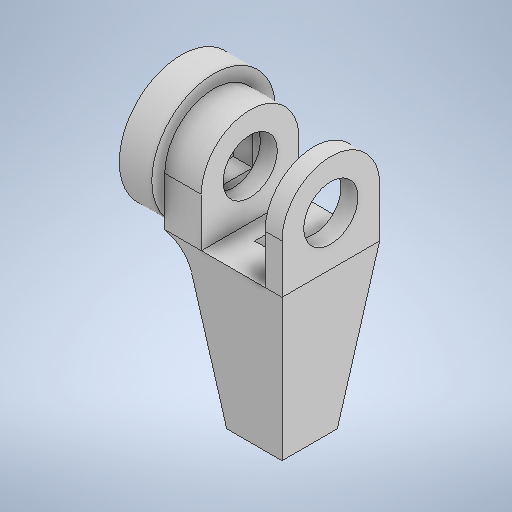
# Autodesk Inventor part: Hip joint 4 med servofeste
Saved by Autodesk Inventor 2025.1 (Build 291241020, 241B)
## iProperties
Created: 2024-10-28
Part Number: Hip joint 4 med servofeste
Material: Generic
Document SubType Name: Modeling
Designer: morte
Density: 1 g/cm^3
Appearance: Default
Author: morte
Autodesk Inventor part; units mm, degrees
ref_plane "YZ Plane" through (0, 0, 0) normal (1, 0, 0) x (0, 1, 0)
ref_plane "XZ Plane" through (0, 0, 0) normal (0, 1, 0) x (-1, 0, 0)
ref_plane "XY Plane" through (0, 0, 0) normal (0, 0, 1) x (1, 0, 0)
sketch "Sketch1" plane through (0, 0, 0) normal (0, 0, 1) x (1, 0, 0)
  line L0 (0, 0) -> (-7.5, 0)
  line L1 (-7.5, 0) -> (-7.5, 15)
  line L2 (-7.5, 15) -> (7.5, 15)
  line L3 (7.5, 15) -> (7.5, 0)
  line L4 (7.5, 0) -> (-7.5, 0)
  dimension "d55" = 7.5
  dimension "d56" = 15
  dimension "d57" = 15
  constraints: 10 end point, 4 perpendicular, 1 horizontal, 1 point on line
  measures "d55" distance of L0.start L0.end
  measures "d56" distance of L0.end L1.end
  measures "d57" distance of L1.end L2.end
extrude "Extrusion1" add sketch "Sketch1" along normal mid plane 15
sketch "Sketch11" plane through (0, 0, 7.5) normal (0, 0, 1) x (1, 0, 0)
  line L0 (7.5, 15) -> (-7.5, 15) projected
  line L1 (0, 15) -> (0, -25)
  line L2 (0, -25) -> (4.25, -25)
  line L3 (0, -25) -> (-4.25, -25)
  line L4 (-7.5, 0) -> (7.5, 0) projected
  line L5 (-4.25, -25) -> (-7.5, 0)
  line L6 (-7.5, 0) -> (7.5, 0)
  line L7 (7.5, 0) -> (4.25, -25)
  point P0 (0, 0)
  dimension "d58" = 40
  dimension "d59" = 4.25
  dimension "d60" = 4.25
  constraints: 12 end point, 2 horizontal, 1 midpoint, 1 parallel, 1 vertical
  measures "d58" distance of L1.start L1.end
  measures "d59" distance of L1.end L2.end
  measures "d60" distance of L1.end L3.end
extrude "Extrusion7" add sketch "Sketch11" against normal blind 15
sketch "Sketch13" plane through (0, 0, 0) normal (1, 0, 0) x (0, 1, 0)
  line L0 (15, -7.5) -> (15, 7.5) projected
  line L1 (15, 0) -> (-25, 0)
  line L2 (-25, 7.5) -> (-25, -7.5) projected
  line L3 (-25, 0) -> (-25, 4.25)
  line L4 (-25, 7.5) -> (-25, -7.5) projected
  line L5 (-25, 4.25) -> (-25, 0)
  line L6 (-25, 0) -> (-25, -4.25)
  line L7 (0, -7.5) -> (15, -7.5) projected
  line L8 (-25, -4.25) -> (0, -7.5)
  line L9 (0, -7.5) -> (0, 7.5)
  line L10 (0, 7.5) -> (-25, 4.25)
  line L11 (-25, 4.25) -> (-25, 7.5)
  line L12 (-25, 7.5) -> (0, 7.5)
  line L13 (-25, -4.25) -> (-25, -7.5)
  line L14 (-25, -7.5) -> (0, -7.5) projected
  line L15 (-25, -7.5) -> (0, -7.5)
  point P0 (0, 0)
  dimension "d68" = 40
  dimension "d69" = 4.25
  dimension "d70" = 4.25
  constraints: 22 end point, 4 collinear, 2 midpoint, 2 point on line, 1 parallel, 1 perpendicular
  measures "d68" distance of L1.start L1.end
  measures "d69" distance of L1.end L3.end
  measures "d70" distance of L1.end L6.end
extrude "Extrusion8" cut sketch "Sketch13" along normal through all both and the other way through all contours L14 L2 L8 | L10 L2 L12
sketch "Sketch15" plane through (-4.25, -25, -4.25) normal (0, -1, 0) x (1, 0, 0)
  line L0 (4.25, 4.25) -> (2.15, 4.25)
  line L1 (0, 8.5) -> (0, 0) projected
  line L2 (2.15, 4.25) -> (2.15, 2.15)
  line L3 (2.15, 2.15) -> (6.35, 2.15)
  line L4 (6.35, 2.15) -> (6.35, 6.35)
  line L5 (6.35, 6.35) -> (2.15, 6.35)
  line L6 (2.15, 6.35) -> (2.15, 4.25)
  point P0 (8.5, 8.5)
  point P1 (8.5, 0)
  dimension "d112" = 2.1
  dimension "d113" = 2.1
  dimension "d114" = 4.2
  dimension "d115" = 4.2
  constraints: 12 end point, 6 perpendicular, 1 point on line
  measures "d112" distance of L0.start L0.end
  measures "d113" distance of L0.end L2.end
  measures "d114" distance of L2.end L3.end
  measures "d115" distance of L3.end L4.end
extrude "Extrusion9" cut sketch "Sketch15" against normal through all
sketch "Sketch16" plane through (0, 0, 7.5) normal (0, 0, 1) x (1, 0, 0)
  line L0 (0, 0) -> (4.9, 0)
  line L1 (-7.5, 0) -> (7.5, 0) projected
  line L2 (4.9, 0) -> (4.9, 16.5506)
  line L3 (0, 0) -> (-4.9, 0)
  line L4 (-4.9, 0) -> (-4.9, 16.5506)
  line L5 (-4.9, 16.5506) -> (4.9, 16.5506)
  dimension "d83" = 4.9
  dimension "d84" = 4.9
  constraints: 10 end point, 2 perpendicular, 2 point on line, 1 vertical
  measures "d83" distance of L0.start L0.end
  measures "d84" distance of L0.start L3.end
extrude "Extrusion10" cut sketch "Sketch16" against normal through all
sketch "Sketch17" plane through (7.5, 15, 7.5) normal (1, 0, 0) x (0, 0, -1)
  line L0 (15, 0) -> (0, 0) projected
  line L1 (0, 0) -> (7.5, 0)
  line L2 (0, 0) -> (0, -15) projected
  line L3 (0, -7.5) -> (0, 0)
  line L4 (0, 0) -> (15, 0)
  line L5 (15, -15) -> (15, 0) projected
  line L6 (15, 0) -> (15, -7.5)
  arc A0 (15, -7.5) -> (0, -7.5) centre (7.5, -7.5) ccw
  line L7 (0, -15) -> (0, 0) projected
  line L8 (0, -7.5) -> (0, 0)
  line L9 (15, 0) -> (0, 0) projected
  line L10 (0, 0) -> (15, 0)
  line L11 (15, 0) -> (15, -7.5)
  point P0 (7.5, -15)
  dimension "d133" = 15
  constraints: 14 end point, 2 horizontal, 2 midpoint, 2 perpendicular, 2 point on circle, 1 centre point, 1 collinear, 1 vertical
  measures "d133" diameter of A0
extrude "Extrusion11" cut sketch "Sketch17" against normal through all
sketch "Sketch18" plane through (7.5, 0, 7.5) normal (1, 0, 0) x (0, 0, -1)
  line L0 (0, 0) -> (0, 15)
  line L1 (0, 15) -> (15, 15)
  line L2 (15, 15) -> (15, 0)
  line L3 (15, 0) -> (0, 0)
  line L4 (0, 15) -> (15, 0)
  line L5 (15, 15) -> (0, 0)
  circle A0 centre (7.5, 7.5) radius 4.15
  point P0 (7.5, 0)
  dimension "d90" = 15
  dimension "d91" = 8.3
  constraints: 12 end point, 4 perpendicular, 1 centre point, 1 midpoint, 1 vertical
  measures "d90" distance of L0.start L0.end
  measures "d91" diameter of A0
extrude "Extrusion12" cut sketch "Sketch18" against normal blind 8.3 contours A0 L4 L5 | L5 L4 A0 | A0 L5 L4 | L4 L5 A0
sketch "Sketch19" plane through (-7.5, 0, -7.5) normal (-1, 0, 0) x (0, 0, 1)
  line L0 (0, 0) -> (0, 15)
  line L1 (0, 15) -> (15, 15)
  line L2 (15, 15) -> (15, 0)
  line L3 (15, 0) -> (0, 0) projected
  line L4 (15, 0) -> (0, 0)
  point P0 (7.5, 0)
  dimension "d94" = 15
  constraints: 8 end point, 3 perpendicular, 1 vertical
  measures "d94" distance of L0.start L0.end
extrude "Extrusion13" add sketch "Sketch19" along normal blind 3
sketch "Sketch20" plane through (-4.9, 0, 7.5) normal (1, 0, 0) x (0, 0, -1)
  line L0 (0, 0) -> (0, 15) projected
  line L1 (0, 0) -> (0, 15)
  line L2 (0, 15) -> (15, 15)
  line L3 (15, 0) -> (0, 0) projected
  line L4 (15, 15) -> (15, 0)
  line L5 (15, 0) -> (0, 0)
  line L6 (0, 0) -> (15, 15)
  line L7 (0, 15) -> (15, 0)
  circle A0 centre (7.5, 7.5) radius 4.15
  point P0 (7.5, 0)
  dimension "d97" = 15
  dimension "d98" = 8.3
  constraints: 12 end point, 2 collinear, 1 centre point, 1 midpoint, 1 perpendicular
  measures "d97" distance of L0.end L2.end
  measures "d98" diameter of A0
extrude "Extrusion14" cut sketch "Sketch20" against normal blind 2.6 contours A0 L7 L6 | L6 L7 A0 | A0 L6 L7 | L7 L6 A0
sketch "Sketch21" plane through (-10.5, 0, -7.5) normal (-1, 0, 0) x (0, 0, 1)
  line L0 (0, 15) -> (0, 0) projected
  line L1 (15, 0) -> (15, 15) projected
  line L2 (0, 0) -> (15, 15)
  line L3 (0, 15) -> (0, 0) projected
  line L4 (15, 15) -> (0, 15)
  line L5 (0, 15) -> (15, 0)
  line L6 (7.5, 7.5) -> (7.5, 10.5)
  line L7 (7.5, 10.5) -> (10.5, 10.5)
  line L8 (10.5, 10.5) -> (10.5, 4.5)
  line L9 (10.5, 4.5) -> (4.5, 4.5)
  line L10 (4.5, 4.5) -> (4.5, 10.5)
  line L11 (4.5, 10.5) -> (10.5, 10.5)
  point P0 (7.5, 0)
  point P1 (0, 7.5)
  dimension "d101" = 3
  dimension "d102" = 3
  dimension "d103" = 6
  dimension "d104" = 6
  constraints: 18 end point, 4 perpendicular, 3 point on line, 1 collinear, 1 midpoint, 1 vertical
  measures "d101" distance of L6.start L6.end
  measures "d102" distance of L6.end L7.end
  measures "d103" distance of L7.end L8.end
  measures "d104" distance of L8.end L9.end
extrude "Extrusion15" cut sketch "Sketch21" against normal blind 3 contours L11 L6 L5 | L5 L2 L10 | L2 L5 L9 | L8 L5 L2 | L2 L6 L7
sketch "Sketch23" plane through (-4.9, 0, 7.5) normal (1, 0, 0) x (0, 0, -1)
  line L0 (0, 0) -> (0, 15) projected
  line L1 (0, 0) -> (0, 15)
  line L2 (0, 15) -> (15, 15)
  line L3 (15, 15) -> (15, 0)
  line L4 (15, 0) -> (0, 0)
  line L5 (0, 15) -> (7.5, 15)
  arc A0 (15, 7.5) -> (0, 7.5) centre (7.5, 7.5) ccw
  line L6 (0, 7.5) -> (0, 15)
  line L7 (15, 15) -> (15, 7.5)
  point P0 (7.5, 0)
  point P1 (0, 7.5)
  dimension "d107" = 15
  constraints: 14 end point, 3 midpoint, 3 perpendicular, 3 point on circle, 1 centre point, 1 collinear, 1 tangent, 1 vertical
  measures "d107" distance of L0.end L2.end
extrude "Extrusion16" cut sketch "Sketch23" against normal through all contours L0 L2 A0 | L2 L3 A0
fillet "Fillet2" radius 5 1 edges at (-7.5, 0, 0)
sketch "Sketch24" plane through (-10.5, 0, -7.5) normal (-1, 0, 0) x (0, 0, 1)
  line L0 (3.25, -25) -> (0, 0) projected
  line L1 (0, 0) -> (7.5, 0)
  line L2 (0, 0) -> (15, 0) projected
  line L3 (7.5, 0) -> (7.5, 4.5)
  line L4 (10.5, 4.5) -> (4.5, 4.5) projected
  line L5 (7.5, 4.5) -> (7.5, 7.5)
  circle A0 centre (7.5, 7.5) radius 9.5
  line L6 (1.669, 0) -> (13.331, 0)
  point P0 (13.331, 0)
  point P1 (1.669, 0)
  dimension "d116" = 3
  dimension "d117" = 19
  constraints: 8 end point, 3 point on line, 2 point on circle, 1 centre point, 1 coincident, 1 collinear, 1 midpoint
  measures "d116" distance of L3.end L5.end
  measures "d117" diameter of A0
extrude "Extrusion17" add sketch "Sketch24" along normal blind 5
sketch "Sketch25" plane through (-15.5, 0, -7.5) normal (-1, 0, 0) x (0, 0, 1)
  line L0 (0, 0) -> (1.669, 0) projected
  line L1 (0, 0) -> (7.5, 0)
  arc A0 (15, 1.669) -> (0, 1.669) centre (7.5, 7.5) ccw projected
  line L2 (7.5, 0) -> (7.5, 7.5)
  line L3 (7.5, 7.5) -> (7.5, 14.5)
  line L4 (7.5, 14.5) -> (9, 14.5)
  circle A1 centre (9, 14.5) radius 0.975
  line L5 (7.5, 7.5) -> (7.5, 0.5)
  line L6 (7.5, 0.5) -> (6, 0.5)
  line L7 (0, 0) -> (15, 0) projected
  circle A2 centre (6, 0.5) radius 0.975
  point P0 (13.331, 0)
  dimension "d120" = 7
  dimension "d121" = 1.5
  dimension "d122" = 1.95
  dimension "d123" = 7
  dimension "d124" = 1.5
  dimension "d125" = 90
  dimension "d126" = 1.95
  constraints: 12 end point, 2 centre point, 2 coincident, 2 horizontal, 1 parallel, 1 perpendicular, 1 point on line, 1 vertical
  measures "d120" distance of L2.end L3.end
  measures "d121" distance of L3.end L4.end
  measures "d122" diameter of A1
  measures "d123" distance of L2.end L5.end
  measures "d124" distance of L5.end L6.end
  measures "d125" angle of L5 L6
  measures "d126" diameter of A2
extrude "Extrusion18" cut sketch "Sketch25" against normal blind 4 contours A2 L1 | L1 A2 | A1
sketch "Sketch26" plane through (-15.5, 7.5, 0) normal (-1, 0, 0) x (0, 0, 1)
  circle A0 centre (0, 0) radius 3
  point P0 (0, -7.5)
  dimension "d129" = 6
  constraints: 1 centre point
  measures "d129" diameter of A0
extrude "Extrusion19" cut sketch "Sketch26" against normal blind 1
equation "\"d92\" = d91"
equation "\"d105\" = d101"
body "Solid1"
